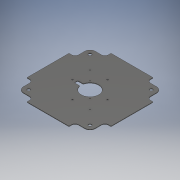
# Autodesk Inventor part: -ZPanel_PCB
Saved by Autodesk Inventor 2018 (Build 220112000, 112)
## iProperties
Created: 2018-11-03
Part Number: -ZPanel_PCB
Material: Epoxy Resin
Document SubType Name: Modeling
Designer: Bradley
Density: 1.14 g/cm^3
Appearance: Smooth - Dark Gray
Mass: 5.79181 g
Surface Area: 172.339 cm^2
Volume: 5.08053 cm^3
Author: Bradley
Autodesk Inventor part; units mm, degrees
ref_plane "YZ Plane" through (0, 0, 0) normal (1, 0, 0) x (0, 1, 0)
ref_plane "XZ Plane" through (0, 0, 0) normal (0, 1, 0) x (-1, 0, 0)
ref_plane "XY Plane" through (0, 0, 0) normal (0, 0, 1) x (1, 0, 0)
sketch "Sketch1" plane through (0, 0, 0) normal (0, 0, 1) x (1, 0, 0)
  line L0 (-48, -48) -> (48, -48)
  line L1 (48, -48) -> (48, 48)
  line L2 (48, 48) -> (-48, 48)
  line L3 (-48, 48) -> (-48, -48)
  line L4 (-48, -48) -> (48, 48) construction
  line L5 (48, -48) -> (-48, 48) construction
  circle A0 centre (0, 0) radius 40 construction
  circle A1 centre (0, 0) radius 10
  line L6 (-9.798, 2) -> (-15, 2)
  arc A2 (-15, 2) -> (-16, 1) centre (-15, 1) ccw
  line L7 (-16, 1) -> (-16, -1)
  arc A3 (-16, -1) -> (-15, -2) centre (-15, -1) ccw
  line L8 (-15, -2) -> (-9.798, -2)
  line L9 (-45, -32.5) -> (45, -32.5) construction
  line L10 (45, -32.5) -> (45, 32.5) construction
  line L11 (45, 32.5) -> (-45, 32.5) construction
  line L12 (-45, 32.5) -> (-45, -32.5) construction
  line L13 (-45, -32.5) -> (45, 32.5) construction
  line L14 (45, -32.5) -> (-45, 32.5) construction
  line L15 (-28, -46.5) -> (28, -46.5) construction
  line L16 (28, -46.5) -> (28, 46.5) construction
  line L17 (28, 46.5) -> (-28, 46.5) construction
  line L18 (-28, 46.5) -> (-28, -46.5) construction
  line L19 (-28, -46.5) -> (28, 46.5) construction
  line L20 (28, -46.5) -> (-28, 46.5) construction
  circle A4 centre (-45, 32.5) radius 4 construction
  circle A5 centre (-28, 46.5) radius 4 construction
  line L21 (-35, -35) -> (35, -35) construction
  line L22 (35, -35) -> (35, 35) construction
  line L23 (35, 35) -> (-35, 35) construction
  line L24 (-35, 35) -> (-35, -35) construction
  line L25 (-35, -35) -> (35, 35) construction
  line L26 (35, -35) -> (-35, 35) construction
  circle A6 centre (-35, 35) radius 3 construction
  line L27 (-24, 48) -> (-24, 45)
  arc A7 (-28, 41) -> (-24, 45) centre (-28, 45) ccw
  line L28 (-28, 41) -> (-35, 41)
  arc A8 (-35, 41) -> (-41, 35) centre (-35, 35) ccw
  line L29 (-41, 35) -> (-41, 28)
  arc A9 (-45, 24) -> (-41, 28) centre (-45, 28) ccw
  line L30 (-45, 24) -> (-48, 24)
  line L31 (48, 24) -> (45, 24)
  arc A10 (41, 28) -> (45, 24) centre (45, 28) ccw
  line L32 (41, 28) -> (41, 35)
  arc A11 (41, 35) -> (35, 41) centre (35, 35) ccw
  line L33 (35, 41) -> (28, 41)
  arc A12 (24, 45) -> (28, 41) centre (28, 45) ccw
  line L34 (24, 45) -> (24, 48)
  line L35 (48, -24) -> (45, -24)
  arc A13 (45, -24) -> (41, -28) centre (45, -28) ccw
  line L36 (41, -28) -> (41, -35)
  arc A14 (35, -41) -> (41, -35) centre (35, -35) ccw
  line L37 (35, -41) -> (28, -41)
  arc A15 (28, -41) -> (24, -45) centre (28, -45) ccw
  line L38 (24, -45) -> (24, -48)
  line L39 (-24, -48) -> (-24, -45)
  arc A16 (-24, -45) -> (-28, -41) centre (-28, -45) ccw
  line L40 (-28, -41) -> (-35, -41)
  arc A17 (-41, -35) -> (-35, -41) centre (-35, -35) ccw
  line L41 (-41, -35) -> (-41, -28)
  arc A18 (-41, -28) -> (-45, -24) centre (-45, -28) ccw
  line L42 (-45, -24) -> (-48, -24)
  dimension "d0" = 96
  dimension "d1" = 96
  dimension "d3" = 80
  dimension "d7" = 20
  dimension "d8" = 1
  dimension "d9" = 4
  dimension "d10" = 16
  dimension "d48" = 90
  dimension "d49" = 65
  dimension "d50" = 56
  dimension "d51" = 93
  dimension "d52" = 8
  dimension "d53" = 70
  dimension "d54" = 6
  dimension "d55" = 24
  dimension "d56" = 24
  dimension "d57" = 4
  dimension "d58" = 41
  constraints: 86 end point, 30 point on circle, 27 tangent, 20 perpendicular, 19 centre point, 12 equal radius, 11 point on line, 8 midpoint, 8 parallel, 7 collinear, 6 horizontal, 5 coincident, 5 equal length, 1 concentric, 1 vertical
  measures "d0" distance of L2.end L1.end
  measures "d1" distance of L1.end L0.end
  measures "d3" diameter of A0
  measures "d7" diameter of A1
  measures "d8" radius of A2
  measures "d9" distance between parallel lines of L8 L6
  measures "d10" distance from line of point (0, 0) L7
  measures "d48" distance of L11.end L10.end
  measures "d49" distance of L10.end L9.end
  measures "d50" distance of L17.end L16.end
  measures "d51" distance of L16.end L15.end
  measures "d52" diameter of A4
  measures "d53" distance of L23.end L22.end
  measures "d54" diameter of A6
  measures "d55" distance from line of point (0, 0) L27
  measures "d56" distance from line of point (0, 0) L30
  measures "d57" radius of A7
  measures "d58" distance from line of point (0, 0) L29
extrude "Extrusion1" add sketch "Sketch1" along normal mid plane 0.6 contours L39 A16 L40 A17 L41 A18 L42 L3 L30 A9 L29 A8 L28 A7 L27 L2 L34 A12 L33 A11 L32 A10 L31 L1 L35 A13 L36 A14 L37 A15 L38 L0
fillet "Fillet1" radius 0.5 10 edges at (-9.798, 2, 0) (-9.798, -2, 0) (-24, -48, 0) (-48, -24, 0) (-48, 24, 0) (-24, 48, 0) (24, 48, 0) (48, 24, 0) (48, -24, 0) (24, -48, 0)
sketch "Sketch2" plane through (0, 0, 0.3) normal (0, 0, 1) x (1, 0, 0)
  line L0 (19.4454, -19.4454) -> (8.8388, -8.8388) construction
  line L1 (-19.4454, 19.4454) -> (-8.8388, 8.8388) construction
  line L2 (-23.5, -48) -> (23.5, -48) projected
  line L3 (48, -23.5) -> (48, 23.5) projected
  line L4 (23.5, 48) -> (-23.5, 48) projected
  line L5 (-48, 23.5) -> (-48, -23.5) projected
  arc A0 (-9.7124, -2.381) -> (-10.198, -2) centre (-10.198, -2.5) ccw projected
  line L6 (-10.198, -2) -> (-15, -2) projected
  arc A1 (-16, -1) -> (-15, -2) centre (-15, -1) ccw projected
  line L7 (-16, -1) -> (-16, 1) projected
  arc A2 (-15, 2) -> (-16, 1) centre (-15, 1) ccw projected
  line L8 (-15, 2) -> (-10.198, 2) projected
  arc A3 (-10.198, 2) -> (-9.7124, 2.381) centre (-10.198, 2.5) ccw projected
  arc A4 (-9.7124, -2.381) -> (-9.7124, 2.381) centre (0, 0) ccw projected
  circle A5 centre (0, 0) radius 12.5 construction
  line L9 (-24, 47.5) -> (-24, 45) projected
  arc A6 (-28, 41) -> (-24, 45) centre (-28, 45) ccw projected
  line L10 (-28, 41) -> (-35, 41) projected
  arc A7 (-35, 41) -> (-41, 35) centre (-35, 35) ccw projected
  line L11 (-41, 35) -> (-41, 28) projected
  arc A8 (-45, 24) -> (-41, 28) centre (-45, 28) ccw projected
  line L12 (-45, 24) -> (-47.5, 24) projected
  line L13 (-47.5, -24) -> (-45, -24) projected
  arc A9 (-41, -28) -> (-45, -24) centre (-45, -28) ccw projected
  line L14 (-41, -28) -> (-41, -35) projected
  arc A10 (-41, -35) -> (-35, -41) centre (-35, -35) ccw projected
  line L15 (-35, -41) -> (-28, -41) projected
  arc A11 (-24, -45) -> (-28, -41) centre (-28, -45) ccw projected
  line L16 (-24, -45) -> (-24, -47.5) projected
  line L17 (24, -47.5) -> (24, -45) projected
  arc A12 (28, -41) -> (24, -45) centre (28, -45) ccw projected
  line L18 (28, -41) -> (35, -41) projected
  arc A13 (35, -41) -> (41, -35) centre (35, -35) ccw projected
  line L19 (41, -35) -> (41, -28) projected
  arc A14 (45, -24) -> (41, -28) centre (45, -28) ccw projected
  line L20 (45, -24) -> (47.5, -24) projected
  line L21 (47.5, 24) -> (45, 24) projected
  arc A15 (41, 28) -> (45, 24) centre (45, 28) ccw projected
  line L22 (41, 28) -> (41, 35) projected
  arc A16 (41, 35) -> (35, 41) centre (35, 35) ccw projected
  line L23 (35, 41) -> (28, 41) projected
  arc A17 (24, 45) -> (28, 41) centre (28, 45) ccw projected
  line L24 (24, 45) -> (24, 47.5) projected
  arc A18 (23.5, -48) -> (24, -47.5) centre (23.5, -47.5) ccw projected
  arc A19 (47.5, -24) -> (48, -23.5) centre (47.5, -23.5) ccw projected
  arc A20 (48, 23.5) -> (47.5, 24) centre (47.5, 23.5) ccw projected
  arc A21 (24, 47.5) -> (23.5, 48) centre (23.5, 47.5) ccw projected
  arc A22 (-23.5, 48) -> (-24, 47.5) centre (-23.5, 47.5) ccw projected
  arc A23 (-47.5, 24) -> (-48, 23.5) centre (-47.5, 23.5) ccw projected
  arc A24 (-48, -23.5) -> (-47.5, -24) centre (-47.5, -23.5) ccw projected
  arc A25 (-24, -47.5) -> (-23.5, -48) centre (-23.5, -47.5) ccw projected
  dimension "d12" = 15
  dimension "d33" = 135
  dimension "d34" = 25
  constraints: 5 coincident, 4 end point, 2 collinear, 2 point on circle, 1 centre point, 1 point on line
  measures "d12" distance of L1.start L1.end
  measures "d33" angle of L2 L1
  measures "d34" diameter of A5
hole "Hole1" at (-8.8388, 8.8388, 0.3) at (-19.4454, 19.4454, 0.3) at (8.8388, -8.8388, 0.3) at (19.4454, -19.4454, 0.3) direction (0, 0, -1) diameter 1 end through all
sketch "Sketch3" plane through (0, 0, 0.3) normal (0, 0, 1) x (1, 0, 0)
  point P0 (0, 0)
  point P1 (-20, 0)
  point P2 (0, -20)
  point P3 (20, 0)
  point P4 (0, 20)
  dimension "d21" = 20
  dimension "d24" = 360
  constraints: 1 horizontal alignment, 5 other
  measures "d21" distance of point (-20, 0) point (0, 0)
hole "Hole2" at (-20, 0, 0.3) at (0, -20, 0.3) at (20, 0, 0.3) at (0, 20, 0.3) direction (0, 0, -1) diameter 1.6 end through all
sketch "Sketch4" plane through (0, 0, 0.3) normal (0, 0, 1) x (1, 0, 0)
  line L0 (-35, -35) -> (35, -35) construction
  line L1 (35, -35) -> (35, 35) construction
  line L2 (35, 35) -> (-35, 35) construction
  line L3 (-35, 35) -> (-35, -35) construction
  line L4 (-35, -35) -> (35, 35) construction
  line L5 (35, -35) -> (-35, 35) construction
  point P0 (0, 0)
  dimension "d35" = 70
  constraints: 12 end point, 4 coincident, 2 midpoint, 2 parallel, 2 perpendicular, 1 horizontal
  measures "d35" distance of L2.end L1.end
hole "Hole3" at (-35, 35, 0.3) at (35, 35, 0.3) at (35, -35, 0.3) at (-35, -35, 0.3) direction (0, 0, -1) diameter 3.4 end through all clearance for "Flat Head Machine Screw" size "M3" standard "Ansi Metric M Profile"
equation "\"d56\" = d55"
body "Solid1"
